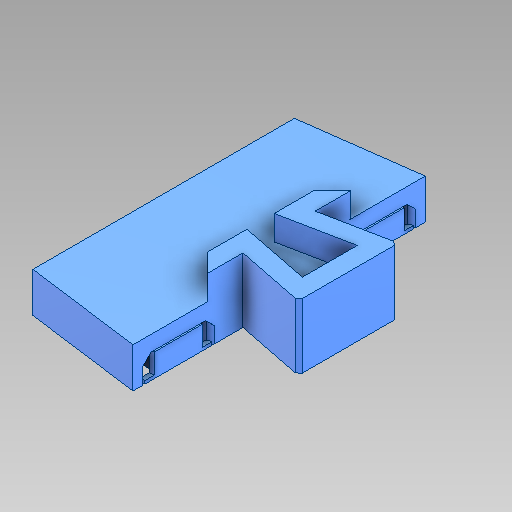
# Autodesk Inventor part: StraightRais-215
Saved by Autodesk Inventor 2021 (Build 250183000, 183)
## iProperties
Created: 2021-02-11
Part Number: StraightRais-215
Material: ABS プラスチック
Document SubType Name: Modeling
Designer: kumagai
Density: 1.06 g/cm^3
Appearance: 滑らか - 青
cp: 0.000 mm
ConnectorLength: 15.000 mm
RailWidth: 38.000 mm
JointFH: 9.500 mm
PrinterOffset: 0.000 mm
StraightLength: 215.000 mm
OuterWall: 2.000 mm
InnerWall: 2.400 mm
InsideWidth: 18.600 mm
RailHeight: 8.400 mm
RailDepth: 3.200 mm
JointMW1: 13.000 mm
JointMW2: 9.400 mm
JointMH: 9.000 mm
JointFW1: 13.300 mm
JointFW2: 9.600 mm
SupportGap: 0.200 mm
SupportRib: 0.500 mm
d71: 5.200 mm
d77: 4.150 mm
Author: kumagai
Autodesk Inventor part; units mm, degrees
ref_plane "YZ Plane" through (0, 0, 0) normal (1, 0, 0) x (0, 1, 0)
ref_plane "XZ Plane" through (0, 0, 0) normal (0, 1, 0) x (-1, 0, 0)
ref_plane "XY Plane" through (0, 0, 0) normal (0, 0, 1) x (1, 0, 0)
sketch "スケッチ1" plane through (0, 0, 0) normal (0, 1, 0) x (-1, 0, 0)
  line L0 (0, -26.6) -> (0, 26.6) projected
  line L1 (-13.8, 0) -> (19.8, 0) projected
  line L2 (0, -4.7) -> (-9, -6.5)
  line L3 (-9, -6.5) -> (-9, 6.5)
  line L4 (-9, 6.5) -> (0, 4.7)
  line L5 (0, -19) -> (0, -4.7)
  line L6 (0, 4.7) -> (0, 19)
  line L7 (2.4, -1.7725) -> (-6.6, -3.5725)
  line L8 (-6.6, -3.5725) -> (-6.6, 3.5725)
  line L9 (-6.6, 3.5725) -> (2.4, 1.7725)
  line L10 (2.4, -6.9) -> (2.4, -1.7725)
  line L11 (2.4, 1.7725) -> (2.4, 6.9)
  line L12 (2.4, -6.9) -> (0, -9.3)
  line L13 (2.4, 6.9) -> (0, 9.3)
  line L14 (15, -17) -> (15, 17)
  line L15 (15, 17) -> (0, 19)
  line L16 (15, -17) -> (0, -19)
  point P0 (0, 0)
  point P1 (0, 9.3)
  point P2 (0, -9.3)
  dimension "d2" = 9
  dimension "d3" = 13
  dimension "d5" = 9.4
  dimension "d13" = 2.4
  dimension "d14" = 2.4
  dimension "d15" = 2.4
  dimension "d24" = 2.4
  dimension "d63" = 2.4
  dimension "d64" = 18.6
  dimension "d65" = 15
  dimension "d74" = 38
  dimension "d75" = 2
  constraints: 30 end point, 3 collinear, 3 parallel, 2 point on line, 2 vertical, 3 other
  measures "d2" distance between parallel lines of L3 L5
  measures "d3" distance of L3.end L2.end
  measures "d5" distance of L4.end L2.start
  measures "d13" distance between parallel lines of L5 L10
  measures "d14" distance between parallel lines of L3 L8
  measures "d15" distance between parallel lines of L4 L9
  measures "d24" distance between parallel lines of L7 L2
  measures "d63" horizontal distance of L12.end L10.start
  measures "d64" distance of L13.end L12.end
  measures "d65" distance between parallel lines of L14 L0
  measures "d74" distance of L5.start L6.end
  measures "d75" vertical distance of L14.end L6.end
extrude "押し出し2" add sketch "スケッチ1" along normal blind 8.4 contours L0 L7 L10 L12 | L2 L3 L1 L8 L7 L0 | L3 L4 L0 L9 L8 L1 | L0 L13 L11 L9
extrude "押し出し1" add sketch "スケッチ1" along normal blind 5.2
sketch "スケッチ2" plane through (0, 0, 0) normal (0, -1, 0) x (1, 0, 0)
  line L0 (0, 125.2612) -> (0, -125.2612) projected
  line L1 (-19.8, 0) -> (13.8, 0) projected
  line L2 (0, 19) -> (0, 4.7) projected
  line L3 (0, -4.7) -> (0, 4.7) projected
  line L4 (-14.95, -6.3) -> (-10.95, -6.3)
  line L5 (-10.95, -6.3) -> (-10.95, -2.6)
  line L6 (-10.95, -2.6) -> (-14.95, -2.6)
  line L7 (-14.95, -2.6) -> (-14.95, -6.3)
  line L8 (-14.95, 2.6) -> (-14.95, 6.3)
  line L9 (-14.95, 6.3) -> (-10.95, 6.3)
  line L10 (-10.95, 6.3) -> (-10.95, 2.6)
  line L11 (-10.95, 2.6) -> (-14.95, 2.6)
  arc A0 (-14.95, -15.85) -> (0, -17.25) centre (0, 63.2723) ccw
  arc A1 (0, -8.95) -> (-14.95, -10.35) centre (0, -89.4723) ccw
  line L12 (-14.95, -15.85) -> (-14.95, -10.35)
  line L13 (0, -17.25) -> (0, -8.95)
  line L14 (0, 8.95) -> (0, 17.25)
  line L15 (-14.95, 10.35) -> (-14.95, 15.85)
  arc A2 (-14.95, 10.35) -> (0, 8.95) centre (0, 89.4723) ccw
  arc A3 (0, 17.25) -> (-14.95, 15.85) centre (0, -63.2723) ccw
  point P0 (0, 17)
  point P1 (0, -17)
  point P2 (0, -17.25)
  point P3 (0, -8.95)
  dimension "d66" = 8.3
  dimension "d67" = 5.5
  dimension "d68" = 17.25
  dimension "d69" = 12.6
  dimension "d70" = 3.7
  dimension "d71" = 5.2
  dimension "d72" = 4
  dimension "d73" = 14.95
  constraints: 24 end point, 8 point on circle, 4 centre point, 4 collinear, 3 parallel, 2 point on line, 2 vertical, 1 equal radius, 1 horizontal, 1 line through centre, 8 other
  measures "d66" distance of L13.end L13.start
  measures "d67" distance of L12.start L12.end
  measures "d68" distance from line of L1 L13.start
  measures "d69" distance between parallel lines of L9 L4
  measures "d70" distance between parallel lines of L9 L11
  measures "d71" distance between parallel lines of L11 L6
  measures "d72" distance between parallel lines of L10 L8
  measures "d73" distance of the line from the sketch origin of L7
extrude "押し出し3" cut sketch "スケッチ2" against normal blind 3.2
chamfer "面取り2" distance 0.6 angle 45 4 edges at (-7.5077, 3.2, 16.8992) (-7.5077, 3.2, 9.3008) (-7.5077, 3.2, -9.3008) (-7.5077, 3.2, -16.8992)
sketch "スケッチ3" plane through (0, 0, 0) normal (0, -1, 0) x (1, 0, 0)
  line L0 (0, 26.6) -> (0, -26.6) projected
  line L1 (1.0922, -13.1) -> (2.1087, -13.1)
  line L2 (0, -9.95) -> (0, -16.25)
  line L3 (0, -16.25) -> (-0.6, -16.25)
  line L4 (-0.6, -16.25) -> (-0.6, -15.5)
  line L5 (-0.6, -15.5) -> (-14.2, -14.6)
  line L6 (-14.2, -14.6) -> (-14.2, -14.0989)
  line L7 (-0.6, -14.9989) -> (-0.6, -13.35)
  line L8 (-0.6, -13.35) -> (-13.1459, -13.35)
  line L9 (-13.1459, -13.35) -> (-13.4654, -14.1475)
  line L10 (-13.4654, -14.1475) -> (-0.6, -14.9989)
  line L11 (-0.6, -12.85) -> (-13.1459, -12.85)
  line L12 (-13.1459, -12.85) -> (-13.4654, -12.0525)
  line L13 (-13.4654, -12.0525) -> (-0.6, -11.2011)
  line L14 (-0.6, -11.2011) -> (-0.6, -12.85)
  line L15 (0, -9.95) -> (-0.6, -9.95)
  line L16 (-0.6, -9.95) -> (-0.6, -10.7)
  line L17 (-0.6, -10.7) -> (-14.2, -11.6)
  line L18 (-14.2, -11.6) -> (-14.2, -12.1011)
  line L19 (-14.2, -12.1011) -> (-13.9, -12.85)
  line L20 (-13.9, -12.85) -> (-13.9, -13.35)
  line L21 (-13.9, -13.35) -> (-14.2, -14.0989)
  line L22 (0, -9.95) -> (0, -8.75)
  line L23 (0, -8.75) -> (-0.3, -8.75)
  line L24 (-0.3, -8.75) -> (-0.6, -9.05)
  line L25 (-0.6, -9.05) -> (-0.6, -9.95)
  line L26 (0, -16.25) -> (0, -17.45)
  line L27 (-0.3, -17.45) -> (-0.6, -17.15)
  line L28 (-0.6, -17.15) -> (-0.6, -16.25)
  line L29 (0, -17.45) -> (-0.3, -17.45)
  point P0 (0, 0)
  point P1 (0, -8.95)
  point P2 (0, -17.25)
  dimension "d76" = 4.15
  dimension "d77" = 4.15
  dimension "d78" = 0.5
  dimension "d79" = 0.6
  dimension "d80" = 14.2
  dimension "d81" = 3
  dimension "d82" = 4.8
  dimension "d83" = 0.3
  dimension "d84" = 0.5
  dimension "d85" = 0.7
  dimension "d86" = 0.2
  dimension "d87" = 45
  dimension "d88" = 0.3
  dimension "d89" = 1
  constraints: 58 end point, 5 horizontal, 5 parallel, 4 point on line, 4 vertical, 3 collinear, 3 perpendicular, 3 symmetric about line, 11 other
  measures "d76" distance from line of L1 point (0, -8.95)
  measures "d77" distance from line of L1 point (0, -17.25)
  measures "d78" distance between parallel lines of L11 L8
  measures "d79" distance of the line from the sketch origin of L14
  measures "d80" distance of the line from the sketch origin of L6
  measures "d81" distance of L17.end L5.end
  measures "d82" distance of L16.end L4.end
  measures "d83" distance between parallel lines of L6 L20
  measures "d84" distance between parallel lines of L5 L10
  measures "d85" distance between parallel lines of L19 L12
  measures "d86" distance from line of L29 point (0, -17.25)
  measures "d87" angle to the sketch x axis of L27
  measures "d88" distance of L26.end L27.start
  measures "d89" distance from line of point (0, -17.25) L3
chamfer "面取り3" distance 0.5 angle 45 6 edges at (0, 1.3, 17.25) (0, 1.3, -8.95) (0, 1.3, -17.25) (9, 4.2, 6.5) (9, 4.2, -6.5) (0, 1.3, 8.95)
extrude "押し出し4" add sketch "スケッチ3" against normal blind 3 contours L0 L3 L4 L5 L6 L21 L20 L19 L18 L17 L16 L15
extrude "押し出し5" add sketch "スケッチ3" against normal blind 0.4 contours L0 L15 L25 L24 L23 | L0 L29 L27 L28 L3
mirror "ミラー5" about plane through (0, 0, 0) normal (0, 0, 1) of "押し出し4", "押し出し5"
equation "\"d2\" = JointMH"
equation "\"d3\" = JointMW1 - 2 * cp"
equation "\"d5\" = JointMW2 - 2 * cp"
equation "\"d13\" = InnerWall"
equation "\"d14\" = InnerWall"
equation "\"d15\" = InnerWall"
equation "\"d24\" = InnerWall"
equation "\"d19\" = RailHeight"
equation "\"d17\" = RailHeight - RailDepth"
equation "\"d33\" = RailDepth"
equation "\"rib\" = 0.5"
equation "\"gap\" = 0.2"
equation "\"JointMH\" = 9"
equation "\"JointMW1\" = 13"
equation "\"cp\" = 0"
equation "\"JointMW2\" = 9.4"
equation "\"InnerWall\" = 2.4"
equation "\"RailHeight\" = 8.4"
equation "\"RailDepth\" = 3.2"
